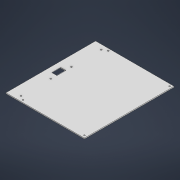
# Autodesk Inventor part: Obenplatte_hinten
Saved by Autodesk Inventor 2021 (Build 250183000, 183)
## iProperties
Created: 2021-02-01
Part Number: Obenplatte_hinten
Material: Generisch
Document SubType Name: Modeling
Designer: laure
Density: 1 g/cm^3
Appearance: Vorgabe
Author: laure
## iProperties of the stored document _3D-Druck.ipt
Created: 2021-02-04
Part Number: _3D-Druck
Material: Generisch
Document SubType Name: Modeling
Designer: Ctroi
Density: 1 g/cm^3
Appearance: Vorgabe
Author: Ctroi
Autodesk Inventor part; units mm, degrees
ref_plane "YZ Plane" through (0, 0, 0) normal (1, 0, 0) x (0, 1, 0)
ref_plane "XZ Plane" through (0, 0, 0) normal (0, 1, 0) x (-1, 0, 0)
ref_plane "XY Plane" through (0, 0, 0) normal (0, 0, 1) x (1, 0, 0)
sketch "Skizze1" plane through (0, 0, 0) normal (0, 1, 0) x (-1, 0, 0)
  line L0 (87.5, -100) -> (-87.5, -100)
  line L1 (-87.5, -100) -> (-87.5, 100)
  line L2 (-87.5, 100) -> (87.5, 100)
  line L3 (87.5, 100) -> (87.5, -100)
  line L4 (0, -140) -> (0, 140) projected
  line L5 (-122.5, 0) -> (122.5, 0) projected
  point P0 (0, 0)
  dimension "d0" = 175
  dimension "d1" = 200
  constraints: 8 end point, 2 parallel, 1 horizontal, 1 perpendicular, 2 other
  measures "d0" distance of L1.end L2.end
  measures "d1" distance of L0.end L1.end
extrude "Extrusion1" add sketch "Skizze1" along normal blind 2
sketch "Skizze2" plane through (0, 2, 0) normal (0, 1, 0) x (1, 0, 0)
  circle A0 centre (-54.5, 95) radius 1.6
  line L0 (0, 140) -> (0, -140) projected
  line L1 (122.5, 0) -> (-122.5, 0) projected
  line L2 (87.5, 100) -> (-87.5, 100) projected
  circle A1 centre (82.5, 95) radius 1.6
  circle A2 centre (-54.5, -95) radius 1.6
  circle A3 centre (82.5, -95) radius 1.6
  line L3 (-87.5, 100) -> (-87.5, -100) projected
  line L4 (87.5, -100) -> (87.5, 100) projected
  point P0 (0, 0)
  dimension "d4" = 3.2
  dimension "d6" = 5
  dimension "d7" = 3.2
  dimension "d9" = 5
  dimension "d40" = 33
  dimension "d41" = 5
  constraints: 4 centre point, 2 symmetric about line, 2 other
  measures "d4" diameter of A0
  measures "d6" distance from line of A0.centre L2
  measures "d7" diameter of A1
  measures "d9" distance from line of L2 A1.centre
  measures "d40" distance from line of L3 A0.centre
  measures "d41" distance from line of L4 A1.centre
extrude "Extrusion2" cut sketch "Skizze2" against normal up to surface (2 mm away) contours A0 | A1 | A2 | A3
sketch "Skizze3" plane through (0, 2, 0) normal (0, 1, 0) x (1, 0, 0)
  line L0 (87.5, -100) -> (87.5, 100) projected
  line L1 (-87.5, -100) -> (87.5, -100) projected
  line L2 (87.5, 100) -> (-87.5, 100) projected
  circle A0 centre (-64.5, 89.5) radius 1.6
  line L3 (-87.5, 100) -> (-87.5, -100) projected
  circle A1 centre (-64.5, 23) radius 1.6
  circle A2 centre (-64.5, -23) radius 1.6
  circle A3 centre (-64.5, -89.5) radius 1.6
  point P0 (0, 0)
  dimension "d26" = 3.2
  dimension "d27" = 23
  dimension "d28" = 10.5
  dimension "d29" = 3.2
  dimension "d30" = 23
  dimension "d31" = 77
  dimension "d32" = 3.2
  dimension "d33" = 23
  dimension "d34" = 77
  dimension "d35" = 3.2
  dimension "d36" = 10.5
  dimension "d37" = 23
  constraints: 4 centre point
  measures "d26" diameter of A0
  measures "d27" distance from line of L3 A0.centre
  measures "d28" distance from line of L2 A0.centre
  measures "d29" diameter of A1
  measures "d30" distance from line of L3 A1.centre
  measures "d31" distance from line of L2 A1.centre
  measures "d32" diameter of A2
  measures "d33" distance from line of L3 A2.centre
  measures "d34" distance from line of L1 A2.centre
  measures "d35" diameter of A3
  measures "d36" distance from line of L1 A3.centre
  measures "d37" distance from line of L3 A3.centre
extrude "Extrusion4" cut sketch "Skizze3" against normal up to surface (2 mm away) contours A0 | A1 | A2 | A3
sketch "Skizze4" plane through (0, 2, 0) normal (0, 1, 0) x (1, 0, 0)
  line L0 (-75.5, -10) -> (-65.5, -10)
  line L1 (-65.5, -10) -> (-65.5, 10)
  line L2 (-65.5, 10) -> (-75.5, 10)
  line L3 (-75.5, 10) -> (-75.5, -10)
  line L4 (-75.5, -10) -> (-65.5, 10) construction
  line L5 (-65.5, -10) -> (-75.5, 10) construction
  line L6 (-87.5, 100) -> (-87.5, -100) projected
  line L7 (87.5, 100) -> (-87.5, 100) projected
  point P0 (0, 0)
  point P1 (-70.5, 0)
  dimension "d42" = 10
  dimension "d43" = 20
  dimension "d44" = 12
  dimension "d45" = 90
  constraints: 12 end point, 2 midpoint, 2 parallel, 1 horizontal, 1 perpendicular
  measures "d42" distance of L2.end L1.end
  measures "d43" distance of L1.end L0.end
  measures "d44" distance between parallel lines of L6 L3
  measures "d45" distance between parallel lines of L7 L2
extrude "Extrusion5" cut sketch "Skizze4" against normal up to surface (2 mm away)
fillet "Rundung1" radius 2 1 edges at (-75.5, 0, 0)
fillet "Rundung2" radius 2 1 edges at (-65.5, 2, 0)
